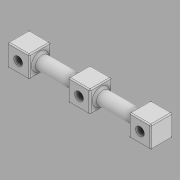
# Autodesk Inventor part: connectingRod
Saved by Autodesk Inventor 2020 (Build 240168000, 168)
## iProperties
Company: Dibujo Computarizado AD2019
Created: 2019-11-16
Part Number: connectingRod
Material: Genérico
Document SubType Name: Modeling
Designer: Gerardo Naranjo
Density: 1 g/cm^3
Appearance: Valor por defecto
Author: Gerardo Naranjo
Title: Connecting Rod
Autodesk Inventor part; units mm, degrees
ref_plane "YZ Plane" through (0, 0, 0) normal (1, 0, 0) x (0, 1, 0)
ref_plane "XZ Plane" through (0, 0, 0) normal (0, 1, 0) x (-1, 0, 0)
ref_plane "XY Plane" through (0, 0, 0) normal (0, 0, 1) x (1, 0, 0)
sketch "Boceto1" plane through (0, 0, 0) normal (0, 0, 1) x (1, 0, 0)
  line L0 (-5, -5) -> (5, -5)
  line L1 (5, -5) -> (5, 5)
  line L2 (5, 5) -> (-5, 5)
  line L3 (-5, 5) -> (-5, -5)
  line L4 (-5, -5) -> (5, 5) construction
  line L5 (5, -5) -> (-5, 5) construction
  circle A0 centre (0, 0) radius 2
  dimension "d0" = 10
  dimension "d1" = 10
  dimension "d2" = 4
  constraints: 12 end point, 2 midpoint, 2 parallel, 1 centre point, 1 coincident, 1 horizontal, 1 perpendicular
  measures "d0" distance of L2.end L1.end
  measures "d1" distance of L1.end L0.end
  measures "d2" diameter of A0
extrude "Extrusión1" add sketch "Boceto1" along normal mid plane 10
sketch "Boceto2" plane through (5, -5, 5) normal (1, 0, 0) x (0, 0, -1)
  circle A0 centre (5, 5) radius 3
  dimension "d5" = 6
  constraints: 1 centre point, 1 coincident
  measures "d5" diameter of A0
extrude "Extrusión2" add sketch "Boceto2" along normal blind 18
sketch "Boceto3" plane through (0, 0, 0) normal (0, 0, 1) x (1, 0, 0)
  line L0 (23, -5) -> (33, -5)
  line L1 (33, -5) -> (33, 5)
  line L2 (33, 5) -> (23, 5)
  line L3 (23, 5) -> (23, -5)
  line L4 (23, -5) -> (33, 5) construction
  line L5 (33, -5) -> (23, 5) construction
  circle A0 centre (28, 0) radius 2
  point P0 (0, 0)
  point P1 (28, 0)
  dimension "d8" = 10
  dimension "d9" = 10
  dimension "d10" = 28
  dimension "d11" = 4
  constraints: 12 end point, 2 midpoint, 2 parallel, 1 centre point, 1 coincident, 1 horizontal, 1 perpendicular
  measures "d8" distance of L2.end L1.end
  measures "d9" distance of L1.end L0.end
  measures "d10" distance of point (28, 0) point (0, 0)
  measures "d11" diameter of A0
extrude "Extrusión3" add sketch "Boceto3" along normal mid plane 10
sketch "Boceto4" plane through (-5, -5, 5) normal (-1, 0, 0) x (0, 0, 1)
  circle A0 centre (-5, 5) radius 3
  dimension "d14" = 6
  constraints: 1 centre point, 1 coincident
  measures "d14" diameter of A0
extrude "Extrusión4" add sketch "Boceto4" along normal blind 18
sketch "Boceto5" plane through (0, 0, 0) normal (0, 0, 1) x (1, 0, 0)
  line L0 (-33, -5) -> (-23, -5)
  line L1 (-23, -5) -> (-23, 5)
  line L2 (-23, 5) -> (-33, 5)
  line L3 (-33, 5) -> (-33, -5)
  line L4 (-33, -5) -> (-23, 5) construction
  line L5 (-23, -5) -> (-33, 5) construction
  circle A0 centre (-28, 0) radius 2
  point P0 (0, 0)
  dimension "d17" = 10
  dimension "d18" = 10
  dimension "d19" = 28
  dimension "d20" = 4
  constraints: 12 end point, 2 midpoint, 2 parallel, 1 centre point, 1 coincident, 1 horizontal, 1 perpendicular
  measures "d17" distance of L2.end L1.end
  measures "d18" distance of L1.end L0.end
  measures "d19" distance of point (0, 0) point (-28, 0)
  measures "d20" diameter of A0
extrude "Extrusión5" add sketch "Boceto5" along normal mid plane 10
fillet "Empalme1" radius 1 4 edges at (-5, 0, -3) (23, 0, 3) (5, 0, 3) (-23, 0, -3)
fillet "Empalme2" radius 0.5 36 edges at (-23, 5, 0) (-28, 5, -5) (-33, 5, 0) (-28, 5, 5) (-23, 0, 5) (-23, 0, -5) (-23, -5, 0) (-28, -5, 5) (-33, 0, 5) (0, 5, 5) (0, 5, -5) (-5, 5, 0) (5, 5, 0) (5, 0, -5) (5, 0, 5) (-5, 0, 5) (0, -5, 5) (5, -5, 0) (28, -5, 5) (33, 0, 5) (33, -5, 0) (33, 0, -5) (28, 5, -5) (33, 5, 0) (23, 5, 0) (23, 0, 5) (28, 5, 5) (23, 0, -5) (23, -5, 0) (-5, 0, -5) (-5, -5, 0) (-33, 0, -5) (-33, -5, 0) (-28, -5, -5) (0, -5, -5) (28, -5, -5)
